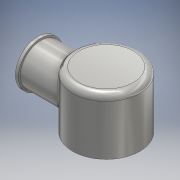
# Autodesk Inventor part: UR5 upper joint shoulder
Saved by Autodesk Inventor 2016 (Build 200138000, 138)
## iProperties
Created: 2017-12-24
Part Number: UR5 upper joint shoulder
Material: Aluminum 6061-AHC
Document SubType Name: Modeling
Designer: kornbot
Density: 2.7 g/cm^3
Appearance: Aluminum - Dark
Author: kornbot
Autodesk Inventor part; units mm, degrees
ref_plane "YZ Plane" through (0, 0, 0) normal (1, 0, 0) x (0, 1, 0)
ref_plane "XZ Plane" through (0, 0, 0) normal (0, 1, 0) x (-1, 0, 0)
ref_plane "XY Plane" through (0, 0, 0) normal (0, 0, 1) x (1, 0, 0)
sketch "Sketch1" plane through (0, 0, 0) normal (0, 0, 1) x (1, 0, 0)
  circle A0 centre (0, 0) radius 43.5575
  circle A1 centre (0, 0) radius 45
  dimension "d0" = 87.115
  dimension "d1" = 90
  constraints: 2 centre point, 2 coincident
  measures "d0" diameter of A0
  measures "d1" diameter of A1
extrude "Extrusion1" add sketch "Sketch1" along normal blind 50.75
sketch "Sketch2" plane through (0, 0, 50.75) normal (0, 0, 1) x (1, 0, 0)
  circle A0 centre (0, 0) radius 45
  constraints: 1 centre point, 1 coincident
extrude "Extrusion2" add sketch "Sketch2" along normal blind 25
fillet "Fillet1" radius 8.5 1 edges at (-45, 0, 75.75)
sketch "Sketch3" plane through (0, 0, 50.75) normal (0, 0, -1) x (-1, 0, 0)
  line L0 (50.9793, -19.9218) -> (46.6884, -19.9218)
  line L1 (46.6884, -19.9218) -> (46.6884, 13.3833)
  line L2 (46.6884, 13.3833) -> (50.9793, 13.3833)
  line L3 (50.9793, 13.3833) -> (50.9793, -19.9218)
  point P0 (0, 0)
  constraints: 8 end point, 2 parallel, 1 horizontal, 1 perpendicular
extrude "Extrusion3" add sketch "Sketch3" along normal blind 25
sketch "Sketch4" plane through (-50.9793, -19.9218, 50.75) normal (-1, 0, 0) x (0, 0, 1)
  line L0 (0, 33.3051) -> (0, 0) projected
  line L1 (0, 33.3051) -> (-25, 0)
  line L2 (-25, 0) -> (0, 0)
  line L3 (0, 0) -> (-25, 33.3051)
  circle A0 centre (-12.5, 16.6526) radius 27.4504
  point P0 (-50.75, 19.9218)
  constraints: 6 end point, 1 centre point, 1 midpoint
extrude "Extrusion4" add sketch "Sketch4" along normal blind 55 contours L0 L3 L1 | L2 L1 L3 | A0
sketch "Sketch5" plane through (-46.6884, -19.9218, 25.75) normal (0, -1, 0) x (1, 0, 0)
  line L0 (0, 25) -> (0, 0) projected
  line L1 (-4.2908, 0) -> (0, 0) projected
  line L2 (0, 25) -> (-4.2908, 25)
  line L3 (-4.2908, 25) -> (-4.2908, 0)
  line L4 (-4.2908, 0) -> (0, 0)
  line L5 (0, 0) -> (0, 25)
  point P0 (46.6884, -25.75)
  constraints: 8 end point, 2 parallel, 1 horizontal, 1 perpendicular
extrude "Extrusion5" cut sketch "Sketch5" against normal blind 101.25
sketch "Sketch6" plane through (-50.9793, -3.2692, 38.25) normal (1, 0, 0) x (0, 0, -1)
  circle A0 centre (0, 0) radius 27.4504
  point P0 (38.25, 3.2692)
  constraints: 1 centre point
extrude "Extrusion6" cut sketch "Sketch6" along normal blind 21.25
sketch "Sketch7" plane through (-105.9793, -3.2692, 38.25) normal (-1, 0, 0) x (0, 0, 1)
  circle A0 centre (0, 0) radius 25.5
  point P0 (-38.25, 3.2692)
  dimension "d15" = 51
  constraints: 1 centre point
  measures "d15" diameter of A0
extrude "Extrusion7" cut sketch "Sketch7" against normal blind 85
sketch "Sketch8" plane through (-50.9793, -3.2692, 38.25) normal (1, 0, 0) x (0, 0, -1)
  arc A0 (-12.5, 22.2261) -> (-12.5, -22.2261) centre (0, 0) ccw projected
  circle A1 centre (0, 0) radius 27.4504
  point P0 (38.25, 3.2692)
  constraints: 1 centre point, 1 coincident
extrude "Extrusion8" add sketch "Sketch8" along normal blind 18.75
sketch "Sketch9" plane through (-50.9793, -3.2692, 38.25) normal (-1, 0, 0) x (0, 0, 1)
  circle A0 centre (0, 0) radius 25.5
  point P0 (-38.25, 3.2692)
  constraints: 1 centre point
extrude "Extrusion9" cut sketch "Sketch9" against normal blind 37.5
sketch "Sketch10" plane through (0, 0, 0) normal (0, 0, -1) x (-1, 0, 0)
  circle A0 centre (0, 0) radius 43.5575 projected
  line L0 (32.2293, 21.17) -> (38.0669, 21.17) projected
  line L1 (31.8887, -29.671) -> (33.7142, -29.671)
  line L2 (33.7142, -29.671) -> (33.7142, 21.17)
  line L3 (33.7142, 21.17) -> (31.8887, 21.17)
  line L4 (31.8887, 21.17) -> (31.8887, -29.671)
  constraints: 8 end point, 2 parallel, 1 horizontal, 1 perpendicular, 1 point on circle, 1 point on line
extrude "Extrusion10" cut sketch "Sketch10" against normal blind 74.25 contours A0 L2 L0 | A0 L4 L3 L0 L2
sketch "Sketch11" plane through (-105.9793, -3.2692, 38.25) normal (-1, 0, 0) x (0, 0, 1)
  circle A0 centre (0, 0) radius 27.4504
  circle A1 centre (0, 0) radius 25.5
  point P0 (-38.25, 3.2692)
  constraints: 2 centre point, 1 coincident
extrude "Extrusion11" cut sketch "Sketch11" against normal blind 17.5
sketch "Sketch12" plane through (-88.4793, -3.2692, 38.25) normal (-1, 0, 0) x (0, 0, 1)
  arc A0 (7.2783, 24.4392) -> (-7.2783, 24.4392) centre (0, 0) ccw projected
  line L0 (0, 25.5) -> (0.7499, 25.489)
  line L1 (0, 25.5) -> (-0.7499, 25.489)
  line L2 (0, 24) -> (0.3, 24)
  line L3 (0.3, 24) -> (0.7499, 25.489)
  line L4 (0, 24) -> (-0.3, 24)
  line L5 (-0.7499, 25.489) -> (-0.3, 24)
  line L6 (-0.7499, 25.489) -> (0.7499, 25.489)
  line L7 (-2.2527, 23.8959) -> (-1.9636, 25.4243)
  line L8 (-2.551, 23.864) -> (-2.2527, 23.8959)
  line L9 (-2.551, 23.864) -> (-2.8493, 23.8321)
  line L10 (-3.455, 25.2649) -> (-2.8493, 23.8321)
  line L11 (-3.455, 25.2649) -> (-1.9636, 25.4243)
  line L12 (-4.78, 23.5211) -> (-4.655, 25.0715)
  line L13 (-5.0732, 23.4577) -> (-4.78, 23.5211)
  line L14 (-5.0732, 23.4577) -> (-5.3664, 23.3943)
  line L15 (-6.1209, 24.7545) -> (-5.3664, 23.3943)
  line L16 (-6.1209, 24.7545) -> (-4.655, 25.0715)
  line L17 (-7.253, 22.8798) -> (-7.2935, 24.4347)
  line L18 (-7.5378, 22.7855) -> (-7.253, 22.8798)
  line L19 (-7.5378, 22.7855) -> (-7.8227, 22.6913)
  line L20 (-8.7175, 23.9636) -> (-7.8227, 22.6913)
  line L21 (-8.7175, 23.9636) -> (-7.2935, 24.4347)
  line L22 (-9.6439, 21.9792) -> (-9.8495, 23.521)
  line L23 (-9.9171, 21.8552) -> (-9.6439, 21.9792)
  line L24 (-9.9171, 21.8552) -> (-10.1903, 21.7313)
  line L25 (-11.2153, 22.9013) -> (-10.1903, 21.7313)
  line L26 (-11.2153, 22.9013) -> (-9.8495, 23.521)
  line L27 (-11.9255, 20.8296) -> (-12.2938, 22.3408)
  line L28 (-12.184, 20.6773) -> (-11.9255, 20.8296)
  line L29 (-12.184, 20.6773) -> (-12.4424, 20.525)
  line L30 (-13.586, 21.5794) -> (-12.4424, 20.525)
  line L31 (-13.586, 21.5794) -> (-12.2938, 22.3408)
  line L32 (-14.072, 19.444) -> (-14.5988, 20.9075)
  line L33 (-14.3128, 19.2651) -> (-14.072, 19.444)
  line L34 (-14.3128, 19.2651) -> (-14.5536, 19.0862)
  line L35 (-15.8028, 20.0131) -> (-14.5536, 19.0862)
  line L36 (-15.8028, 20.0131) -> (-14.5988, 20.9075)
  line L37 (-16.0591, 17.8381) -> (-16.7384, 19.2373)
  line L38 (-16.2795, 17.6346) -> (-16.0591, 17.8381)
  line L39 (-16.2795, 17.6346) -> (-16.4999, 17.4311)
  line L40 (-17.8405, 18.22) -> (-16.4999, 17.4311)
  line L41 (-17.8405, 18.22) -> (-16.7384, 19.2373)
  line L42 (-17.8641, 16.03) -> (-18.6884, 17.3491)
  line L43 (-18.0617, 15.8043) -> (-17.8641, 16.03)
  line L44 (-18.0617, 15.8043) -> (-18.2593, 15.5785)
  line L45 (-19.6761, 16.2204) -> (-18.2593, 15.5785)
  line L46 (-19.6761, 16.2204) -> (-18.6884, 17.3491)
  line L47 (-19.4668, 14.0404) -> (-20.4267, 15.2644)
  line L48 (-19.6393, 13.7949) -> (-19.4668, 14.0404)
  line L49 (-19.6393, 13.7949) -> (-19.8117, 13.5494)
  line L50 (-21.2887, 14.0371) -> (-19.8117, 13.5494)
  line L51 (-21.2887, 14.0371) -> (-20.4267, 15.2644)
  line L52 (-20.8489, 11.8916) -> (-21.9334, 13.0067)
  line L53 (-20.9943, 11.6292) -> (-20.8489, 11.8916)
  line L54 (-20.9943, 11.6292) -> (-21.1397, 11.3668)
  line L55 (-22.6602, 11.6947) -> (-21.1397, 11.3668)
  line L56 (-22.6602, 11.6947) -> (-21.9334, 13.0067)
  line L57 (-21.9948, 9.6082) -> (-23.1917, 10.6016)
  line L58 (-22.1115, 9.3318) -> (-21.9948, 9.6082)
  line L59 (-22.1115, 9.3318) -> (-22.2281, 9.0554)
  line L60 (-23.7749, 9.2198) -> (-22.2281, 9.0554)
  line L61 (-23.7749, 9.2198) -> (-23.1917, 10.6016)
  line L62 (-22.8915, 7.2158) -> (-24.1872, 8.0764)
  line L63 (-22.9781, 6.9286) -> (-22.8915, 7.2158)
  line L64 (-22.9781, 6.9286) -> (-23.0647, 6.6414)
  line L65 (-24.6202, 6.6405) -> (-23.0647, 6.6414)
  line L66 (-24.6202, 6.6405) -> (-24.1872, 8.0764)
  line L67 (-23.5288, 4.7417) -> (-24.9087, 5.4598)
  line L68 (-23.5844, 4.4469) -> (-23.5288, 4.7417)
  line L69 (-23.5844, 4.4469) -> (-23.64, 4.1521)
  line L70 (-25.1866, 3.9859) -> (-23.64, 4.1521)
  line L71 (-25.1866, 3.9859) -> (-24.9087, 5.4598)
  line L72 (-23.8996, 2.2139) -> (-25.3479, 2.7812)
  line L73 (-23.9235, 1.9149) -> (-23.8996, 2.2139)
  line L74 (-23.9235, 1.9149) -> (-23.9474, 1.6158)
  line L75 (-25.4675, 1.2861) -> (-23.9474, 1.6158)
  line L76 (-25.4675, 1.2861) -> (-25.3479, 2.7812)
  line L77 (-23.9995, -0.339) -> (-25.4999, 0.0711)
  line L78 (-23.9915, -0.6389) -> (-23.9995, -0.339)
  line L79 (-23.9915, -0.6389) -> (-23.9835, -0.9388)
  line L80 (-25.46, -1.4282) -> (-23.9835, -0.9388)
  line L81 (-25.46, -1.4282) -> (-25.4999, 0.0711)
  line L82 (-23.8275, -2.8881) -> (-25.363, -2.6398)
  line L83 (-23.7877, -3.1854) -> (-23.8275, -2.8881)
  line L84 (-23.7877, -3.1854) -> (-23.7479, -3.4828)
  line L85 (-25.1639, -4.1263) -> (-23.7479, -3.4828)
  line L86 (-25.1639, -4.1263) -> (-25.363, -2.6398)
  line L87 (-23.3855, -5.4044) -> (-24.9387, -5.3207)
  line L88 (-23.3143, -5.6958) -> (-23.3855, -5.4044)
  line L89 (-23.3143, -5.6958) -> (-23.2431, -5.9873)
  line L90 (-24.5828, -6.7777) -> (-23.2431, -5.9873)
  line L91 (-24.5828, -6.7777) -> (-24.9387, -5.3207)
  line L92 (-22.6786, -7.8595) -> (-24.2319, -7.9414)
  line L93 (-22.5768, -8.1417) -> (-22.6786, -7.8595)
  line L94 (-22.5768, -8.1417) -> (-22.475, -8.4239)
  line L95 (-23.7231, -9.3523) -> (-22.475, -8.4239)
  line L96 (-23.7231, -9.3523) -> (-24.2319, -7.9414)
  line L97 (-21.7147, -10.2256) -> (-23.2505, -10.4721)
  line L98 (-21.5835, -10.4954) -> (-21.7147, -10.2256)
  line L99 (-21.5835, -10.4954) -> (-21.4523, -10.7652)
  line L100 (-22.5946, -11.8209) -> (-21.4523, -10.7652)
  line L101 (-22.5946, -11.8209) -> (-23.2505, -10.4721)
  line L102 (-20.5048, -12.4758) -> (-22.0057, -12.8842)
  line L103 (-20.3456, -12.7301) -> (-20.5048, -12.4758)
  line L104 (-20.3456, -12.7301) -> (-20.1865, -12.9844)
  line L105 (-21.2101, -14.1556) -> (-20.1865, -12.9844)
  line L106 (-21.2101, -14.1556) -> (-22.0057, -12.8842)
  line L107 (-19.0625, -14.5846) -> (-20.5115, -15.1502)
  line L108 (-18.8772, -14.8206) -> (-19.0625, -14.5846)
  line L109 (-18.8772, -14.8206) -> (-18.692, -15.0566)
  line L110 (-19.5853, -16.3299) -> (-18.692, -15.0566)
  line L111 (-19.5853, -16.3299) -> (-20.5115, -15.1502)
  line L112 (-17.4043, -16.5282) -> (-18.7849, -17.2446)
  line L113 (-17.195, -16.7432) -> (-17.4043, -16.5282)
  line L114 (-17.195, -16.7432) -> (-16.9857, -16.9581)
  line L115 (-17.7386, -18.3192) -> (-16.9857, -16.9581)
  line L116 (-17.7386, -18.3192) -> (-18.7849, -17.2446)
  line L117 (-15.5488, -18.2845) -> (-16.8455, -19.1436)
  line L118 (-15.3179, -18.476) -> (-15.5488, -18.2845)
  line L119 (-15.3179, -18.476) -> (-15.0869, -18.6675)
  line L120 (-15.6909, -20.1009) -> (-15.0869, -18.6675)
  line L121 (-15.6909, -20.1009) -> (-16.8455, -19.1436)
  line L122 (-13.5172, -19.8337) -> (-14.7152, -20.8258)
  line L123 (-13.2672, -19.9995) -> (-13.5172, -19.8337)
  line L124 (-13.2672, -19.9995) -> (-13.0172, -20.1654)
  line L125 (-13.4654, -21.6549) -> (-13.0172, -20.1654)
  line L126 (-13.4654, -21.6549) -> (-14.7152, -20.8258)
  line L127 (-11.3324, -21.1581) -> (-12.4182, -22.2719)
  line L128 (-11.0662, -21.2964) -> (-11.3324, -21.1581)
  line L129 (-11.0662, -21.2964) -> (-10.8, -21.4348)
  line L130 (-11.0873, -22.9635) -> (-10.8, -21.4348)
  line L131 (-11.0873, -22.9635) -> (-12.4182, -22.2719)
  line L132 (-9.0193, -22.2428) -> (-9.9805, -23.4657)
  line L133 (-8.7399, -22.3521) -> (-9.0193, -22.2428)
  line L134 (-8.7399, -22.3521) -> (-8.4605, -22.4613)
  line L135 (-8.5837, -24.0119) -> (-8.4605, -22.4613)
  line L136 (-8.5837, -24.0119) -> (-9.9805, -23.4657)
  line L137 (-6.6039, -23.0755) -> (-7.4297, -24.3936)
  line L138 (-6.3145, -23.1544) -> (-6.6039, -23.0755)
  line L139 (-6.3145, -23.1544) -> (-6.025, -23.2334)
  line L140 (-5.9827, -24.7882) -> (-6.025, -23.2334)
  line L141 (-5.9827, -24.7882) -> (-7.4297, -24.3936)
  line L142 (-4.1137, -23.6467) -> (-4.7947, -25.0452)
  line L143 (-3.8175, -23.6944) -> (-4.1137, -23.6467)
  line L144 (-3.8175, -23.6944) -> (-3.5213, -23.7422)
  line L145 (-3.314, -25.2837) -> (-3.5213, -23.7422)
  line L146 (-3.314, -25.2837) -> (-4.7947, -25.0452)
  line L147 (-1.5769, -23.95) -> (-2.1054, -25.4129)
  line L148 (-1.2773, -23.966) -> (-1.5769, -23.95)
  line L149 (-1.2773, -23.966) -> (-0.9778, -23.982)
  line L150 (-0.6077, -25.4928) -> (-0.9778, -23.982)
  line L151 (-0.6077, -25.4928) -> (-2.1054, -25.4129)
  line L152 (0.9778, -23.982) -> (0.6077, -25.4928)
  line L153 (1.2773, -23.966) -> (0.9778, -23.982)
  line L154 (1.2773, -23.966) -> (1.5769, -23.95)
  line L155 (2.1054, -25.4129) -> (1.5769, -23.95)
  line L156 (2.1054, -25.4129) -> (0.6077, -25.4928)
  line L157 (3.5213, -23.7422) -> (3.314, -25.2837)
  line L158 (3.8175, -23.6944) -> (3.5213, -23.7422)
  line L159 (3.8175, -23.6944) -> (4.1137, -23.6467)
  line L160 (4.7947, -25.0452) -> (4.1137, -23.6467)
  line L161 (4.7947, -25.0452) -> (3.314, -25.2837)
  line L162 (6.025, -23.2334) -> (5.9827, -24.7882)
  line L163 (6.3145, -23.1544) -> (6.025, -23.2334)
  line L164 (6.3145, -23.1544) -> (6.6039, -23.0755)
  line L165 (7.4297, -24.3936) -> (6.6039, -23.0755)
  line L166 (7.4297, -24.3936) -> (5.9827, -24.7882)
  line L167 (8.4605, -22.4613) -> (8.5837, -24.0119)
  line L168 (8.7399, -22.3521) -> (8.4605, -22.4613)
  line L169 (8.7399, -22.3521) -> (9.0193, -22.2428)
  line L170 (9.9805, -23.4657) -> (9.0193, -22.2428)
  line L171 (9.9805, -23.4657) -> (8.5837, -24.0119)
  line L172 (10.8, -21.4348) -> (11.0873, -22.9635)
  line L173 (11.0662, -21.2964) -> (10.8, -21.4348)
  line L174 (11.0662, -21.2964) -> (11.3324, -21.1581)
  line L175 (12.4182, -22.2719) -> (11.3324, -21.1581)
  line L176 (12.4182, -22.2719) -> (11.0873, -22.9635)
  line L177 (13.0172, -20.1654) -> (13.4654, -21.6549)
  line L178 (13.2672, -19.9995) -> (13.0172, -20.1654)
  line L179 (13.2672, -19.9995) -> (13.5172, -19.8337)
  line L180 (14.7152, -20.8258) -> (13.5172, -19.8337)
  line L181 (14.7152, -20.8258) -> (13.4654, -21.6549)
  line L182 (15.0869, -18.6675) -> (15.6909, -20.1009)
  line L183 (15.3179, -18.476) -> (15.0869, -18.6675)
  line L184 (15.3179, -18.476) -> (15.5488, -18.2845)
  line L185 (16.8455, -19.1436) -> (15.5488, -18.2845)
  line L186 (16.8455, -19.1436) -> (15.6909, -20.1009)
  line L187 (16.9857, -16.9581) -> (17.7386, -18.3192)
  line L188 (17.195, -16.7432) -> (16.9857, -16.9581)
  line L189 (17.195, -16.7432) -> (17.4043, -16.5282)
  line L190 (18.7849, -17.2446) -> (17.4043, -16.5282)
  line L191 (18.7849, -17.2446) -> (17.7386, -18.3192)
  line L192 (18.692, -15.0566) -> (19.5853, -16.3299)
  line L193 (18.8772, -14.8206) -> (18.692, -15.0566)
  line L194 (18.8772, -14.8206) -> (19.0625, -14.5846)
  line L195 (20.5115, -15.1502) -> (19.0625, -14.5846)
  line L196 (20.5115, -15.1502) -> (19.5853, -16.3299)
  line L197 (20.1865, -12.9844) -> (21.2101, -14.1556)
  line L198 (20.3456, -12.7301) -> (20.1865, -12.9844)
  line L199 (20.3456, -12.7301) -> (20.5048, -12.4758)
  line L200 (22.0057, -12.8842) -> (20.5048, -12.4758)
  line L201 (22.0057, -12.8842) -> (21.2101, -14.1556)
  line L202 (21.4523, -10.7652) -> (22.5946, -11.8209)
  line L203 (21.5835, -10.4954) -> (21.4523, -10.7652)
  line L204 (21.5835, -10.4954) -> (21.7147, -10.2256)
  line L205 (23.2505, -10.4721) -> (21.7147, -10.2256)
  line L206 (23.2505, -10.4721) -> (22.5946, -11.8209)
  line L207 (22.475, -8.4239) -> (23.7231, -9.3523)
  line L208 (22.5768, -8.1417) -> (22.475, -8.4239)
  line L209 (22.5768, -8.1417) -> (22.6786, -7.8595)
  line L210 (24.2319, -7.9414) -> (22.6786, -7.8595)
  line L211 (24.2319, -7.9414) -> (23.7231, -9.3523)
  line L212 (23.2431, -5.9873) -> (24.5828, -6.7777)
  line L213 (23.3143, -5.6958) -> (23.2431, -5.9873)
  line L214 (23.3143, -5.6958) -> (23.3855, -5.4044)
  line L215 (24.9387, -5.3207) -> (23.3855, -5.4044)
  line L216 (24.9387, -5.3207) -> (24.5828, -6.7777)
  line L217 (23.7479, -3.4828) -> (25.1639, -4.1263)
  line L218 (23.7877, -3.1854) -> (23.7479, -3.4828)
  line L219 (23.7877, -3.1854) -> (23.8275, -2.8881)
  line L220 (25.363, -2.6398) -> (23.8275, -2.8881)
  line L221 (25.363, -2.6398) -> (25.1639, -4.1263)
  line L222 (23.9835, -0.9388) -> (25.46, -1.4282)
  line L223 (23.9915, -0.6389) -> (23.9835, -0.9388)
  line L224 (23.9915, -0.6389) -> (23.9995, -0.339)
  line L225 (25.4999, 0.0711) -> (23.9995, -0.339)
  line L226 (25.4999, 0.0711) -> (25.46, -1.4282)
  line L227 (23.9474, 1.6158) -> (25.4675, 1.2861)
  line L228 (23.9235, 1.9149) -> (23.9474, 1.6158)
  line L229 (23.9235, 1.9149) -> (23.8996, 2.2139)
  line L230 (25.3479, 2.7812) -> (23.8996, 2.2139)
  line L231 (25.3479, 2.7812) -> (25.4675, 1.2861)
  line L232 (23.64, 4.1521) -> (25.1866, 3.9859)
  line L233 (23.5844, 4.4469) -> (23.64, 4.1521)
  line L234 (23.5844, 4.4469) -> (23.5288, 4.7417)
  line L235 (24.9087, 5.4598) -> (23.5288, 4.7417)
  line L236 (24.9087, 5.4598) -> (25.1866, 3.9859)
  line L237 (23.0647, 6.6414) -> (24.6202, 6.6405)
  line L238 (22.9781, 6.9286) -> (23.0647, 6.6414)
  line L239 (22.9781, 6.9286) -> (22.8915, 7.2158)
  line L240 (24.1872, 8.0764) -> (22.8915, 7.2158)
  line L241 (24.1872, 8.0764) -> (24.6202, 6.6405)
  line L242 (22.2281, 9.0554) -> (23.7749, 9.2198)
  line L243 (22.1115, 9.3318) -> (22.2281, 9.0554)
  line L244 (22.1115, 9.3318) -> (21.9948, 9.6082)
  line L245 (23.1917, 10.6016) -> (21.9948, 9.6082)
  line L246 (23.1917, 10.6016) -> (23.7749, 9.2198)
  line L247 (21.1397, 11.3668) -> (22.6602, 11.6947)
  line L248 (20.9943, 11.6292) -> (21.1397, 11.3668)
  line L249 (20.9943, 11.6292) -> (20.8489, 11.8916)
  line L250 (21.9334, 13.0067) -> (20.8489, 11.8916)
  line L251 (21.9334, 13.0067) -> (22.6602, 11.6947)
  line L252 (19.8117, 13.5494) -> (21.2887, 14.0371)
  line L253 (19.6393, 13.7949) -> (19.8117, 13.5494)
  line L254 (19.6393, 13.7949) -> (19.4668, 14.0404)
  line L255 (20.4267, 15.2644) -> (19.4668, 14.0404)
  line L256 (20.4267, 15.2644) -> (21.2887, 14.0371)
  line L257 (18.2593, 15.5785) -> (19.6761, 16.2204)
  line L258 (18.0617, 15.8043) -> (18.2593, 15.5785)
  line L259 (18.0617, 15.8043) -> (17.8641, 16.03)
  line L260 (18.6884, 17.3491) -> (17.8641, 16.03)
  line L261 (18.6884, 17.3491) -> (19.6761, 16.2204)
  line L262 (16.4999, 17.4311) -> (17.8405, 18.22)
  line L263 (16.2795, 17.6346) -> (16.4999, 17.4311)
  line L264 (16.2795, 17.6346) -> (16.0591, 17.8381)
  line L265 (16.7384, 19.2373) -> (16.0591, 17.8381)
  line L266 (16.7384, 19.2373) -> (17.8405, 18.22)
  line L267 (14.5536, 19.0862) -> (15.8028, 20.0131)
  line L268 (14.3128, 19.2651) -> (14.5536, 19.0862)
  line L269 (14.3128, 19.2651) -> (14.072, 19.444)
  line L270 (14.5988, 20.9075) -> (14.072, 19.444)
  line L271 (14.5988, 20.9075) -> (15.8028, 20.0131)
  line L272 (12.4424, 20.525) -> (13.586, 21.5794)
  line L273 (12.184, 20.6773) -> (12.4424, 20.525)
  line L274 (12.184, 20.6773) -> (11.9255, 20.8296)
  line L275 (12.2938, 22.3408) -> (11.9255, 20.8296)
  line L276 (12.2938, 22.3408) -> (13.586, 21.5794)
  line L277 (10.1903, 21.7313) -> (11.2153, 22.9013)
  line L278 (9.9171, 21.8552) -> (10.1903, 21.7313)
  line L279 (9.9171, 21.8552) -> (9.6439, 21.9792)
  line L280 (9.8495, 23.521) -> (9.6439, 21.9792)
  line L281 (9.8495, 23.521) -> (11.2153, 22.9013)
  line L282 (7.8227, 22.6913) -> (8.7175, 23.9636)
  line L283 (7.5378, 22.7855) -> (7.8227, 22.6913)
  line L284 (7.5378, 22.7855) -> (7.253, 22.8798)
  line L285 (7.2935, 24.4347) -> (7.253, 22.8798)
  line L286 (7.2935, 24.4347) -> (8.7175, 23.9636)
  line L287 (5.3664, 23.3943) -> (6.1209, 24.7545)
  line L288 (5.0732, 23.4577) -> (5.3664, 23.3943)
  line L289 (5.0732, 23.4577) -> (4.78, 23.5211)
  line L290 (4.655, 25.0715) -> (4.78, 23.5211)
  line L291 (4.655, 25.0715) -> (6.1209, 24.7545)
  line L292 (2.8493, 23.8321) -> (3.455, 25.2649)
  line L293 (2.551, 23.864) -> (2.8493, 23.8321)
  line L294 (2.551, 23.864) -> (2.2527, 23.8959)
  line L295 (1.9636, 25.4243) -> (2.2527, 23.8959)
  line L296 (1.9636, 25.4243) -> (3.455, 25.2649)
  point P0 (-38.25, 3.2692)
  dimension "d27" = 0.75
  dimension "d29" = 0.75
  dimension "d30" = 1.5
  dimension "d31" = 0.3
  dimension "d32" = 0.3
  dimension "d35" = 360
  constraints: 594 end point, 59 point on line, 3 point on circle, 591 other
  measures "d27" distance of L0.start L0.end
  measures "d29" distance of L0.start L1.end
  measures "d30" distance of L0.start L2.start
  measures "d31" distance of L2.start L2.end
  measures "d32" distance of L2.start L4.end
extrude "Extrusion12" add sketch "Sketch12" against normal blind 24.25 contours L12 L13 L14 L15 L16 | L7 L8 L9 L10 L11 | L3 L2 L4 L5 L6 | L292 L293 L294 L295 L296 | L287 L288 L289 L290 L291 | L18 L19 L20 L21 L17 | L23 L24 L25 L26 L22 | L28 L29 L30 L31 L27 | L33 L34 L35 L36 L32 | L38 L39 L40 L41 L37 | L43 L44 L45 L46 L42 | L48 L49 L50 L51 L47 | L53 L54 L55 L56 L52 | L58 L59 L60 L61 L57 | L63 L64 L65 L66 L62 | L68 L69 L70 L71 L67 | L73 L74 L75 L76 L72 | L78 L79 L80 L81 L77 | L83 L84 L85 L86 L82 | L88 L89 L90 L91 L87 | L93 L94 L95 L96 L92 | L98 L99 L100 L101 L97 | L103 L104 L105 L106 L102 | L108 L109 L110 L111 L107 | L113 L114 L115 L116 L112 | L118 L119 L120 L121 L117 | L123 L124 L125 L126 L122 | L128 L129 L130 L131 L127 | L133 L134 L135 L136 L132 | L138 L139 L140 L141 L137 | L143 L144 L145 L146 L142 | L148 L149 L150 L151 L147 | L153 L154 L155 L156 L152 | L158 L159 L160 L161 L157 | L163 L164 L165 L166 L162 | L168 L169 L170 L171 L167 | L173 L174 L175 L176 L172 | L178 L179 L180 L181 L177 | L183 L184 L185 L186 L182 | L188 L189 L190 L191 L187 | L193 L194 L195 L196 L192 | L198 L199 L200 L201 L197 | L203 L204 L205 L206 L202 | L208 L209 L210 L211 L207 | L213 L214 L215 L216 L212 | L218 L219 L220 L221 L217 | L223 L224 L225 L226 L222 | L228 L229 L230 L231 L227 | L233 L234 L235 L236 L232 | L238 L239 L240 L241 L237 | L243 L244 L245 L246 L242 | L248 L249 L250 L251 L247 | L253 L254 L255 L256 L252 | L258 L259 L260 L261 L257 | L263 L264 L265 L266 L262 | L268 L269 L270 L271 L267 | L273 L274 L275 L276 L272 | L278 L279 L280 L281 L277 | L283 L284 L285 L286 L282
chamfer "Chamfer1" distance 2 angle 45 1 edges at (-44.7171, -5.038, 65.6434)
sketch "Sketch13" plane through (-88.4793, -3.2692, 38.25) normal (-1, 0, 0) x (0, 0, 1)
  circle A0 centre (0, 0) radius 30
  circle A1 centre (0, 0) radius 27.4504
  point P0 (-38.25, 3.2692)
  dimension "d42" = 60
  constraints: 2 centre point, 1 coincident
  measures "d42" diameter of A0
extrude "Extrusion13" add sketch "Sketch13" against normal blind 4
body "Solid1"
